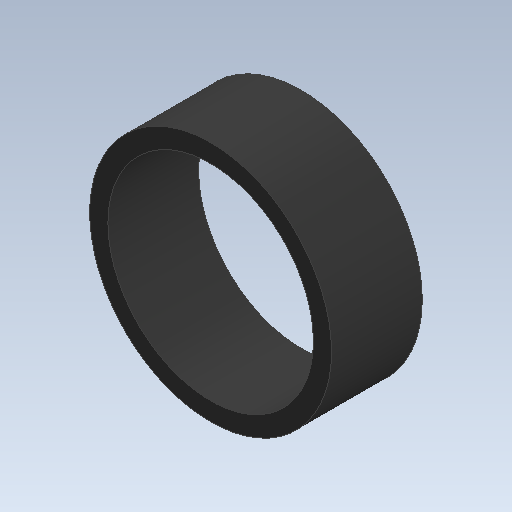
# Autodesk Inventor part: WCP-0075-tread
Saved by Autodesk Inventor 2020 (Build 240168000, 168)
## iProperties
Created: 2022-01-10
Part Number: WCP-0075-tread
Material: Rubber
Document SubType Name: Modeling
Designer: 23kaltomare
Density: 0.93 g/cm^3
Appearance: Rubber - Black
Mass: 79.7165 g
Surface Area: 269.974 cm^2
Volume: 85.7167 cm^3
Author: 23kaltomare
Autodesk Inventor part; units mm, degrees
ref_plane "YZ Plane" through (0, 0, 0) normal (1, 0, 0) x (0, 1, 0)
ref_plane "XZ Plane" through (0, 0, 0) normal (0, 1, 0) x (-1, 0, 0)
ref_plane "XY Plane" through (0, 0, 0) normal (0, 0, 1) x (1, 0, 0)
sketch "Sketch1" plane through (0, 0, 0) normal (0, 0, 1) x (1, 0, 0)
  circle A0 centre (0, 0) radius 43.18
  circle A1 centre (0, 0) radius 50.8
  dimension "d0" = 86.36
  dimension "d1" = 101.6
  constraints: 2 centre point, 2 coincident
  measures "d0" diameter of A0
  measures "d1" diameter of A1
extrude "Extrusion1" add sketch "Sketch1" along normal blind 38.1
body "Solid1"
